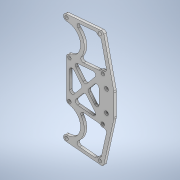
# Autodesk Inventor part: Knee_side_frame
Saved by Autodesk Inventor 2020.4 (Build 244396000, 396)
## iProperties
Created: 2021-09-05
Part Number: Knee_side_frame
Material: アルミニウム 2014-T4
Document SubType Name: Modeling
Designer: masato
Density: 2.8 g/cm^3
Appearance: 滑らか - 淡い灰色
Mass: 7.90232 g
Surface Area: 42.4892 cm^2
Volume: 2.82226 cm^3
Author: masato
Autodesk Inventor part; units mm, degrees
ref_plane "YZ Plane" through (0, 0, 0) normal (1, 0, 0) x (0, 1, 0)
ref_plane "XZ Plane" through (0, 0, 0) normal (0, 1, 0) x (-1, 0, 0)
ref_plane "XY Plane" through (0, 0, 0) normal (0, 0, 1) x (1, 0, 0)
sketch "スケッチ1" plane through (0, 0, 0) normal (0, 0, 1) x (1, 0, 0)
  line L0 (-32.2352, 43.3932) -> (10.6011, 47.1409) construction
  line L1 (10.6011, 47.1409) -> (13.3901, 15.2627) construction
  line L2 (13.3901, 15.2627) -> (-29.4462, 11.515) construction
  line L3 (-29.4462, 11.515) -> (-32.2352, 43.3932) construction
  line L4 (-32.2352, 43.3932) -> (13.3901, 15.2627) construction
  line L5 (10.6011, 47.1409) -> (-29.4462, 11.515) construction
  line L6 (-30.8407, 27.4541) -> (11.9956, 31.2018) construction
  line L7 (7.8305, 44.389) -> (-19.0668, 42.0358) construction
  line L8 (-19.0668, 42.0358) -> (-16.7136, 15.1385) construction
  line L9 (-16.7136, 15.1385) -> (10.1837, 17.4917) construction
  line L10 (10.1837, 17.4917) -> (7.8305, 44.389) construction
  line L11 (7.8305, 44.389) -> (-16.7136, 15.1385) construction
  line L12 (-19.0668, 42.0358) -> (10.1837, 17.4917) construction
  circle A0 centre (-18.8864, 28.5) radius 10.5 construction
  circle A1 centre (-19.0668, 42.0358) radius 1.35
  line L13 (-5.6182, 43.2124) -> (-3.265, 16.3151) construction
  circle A2 centre (7.8305, 44.389) radius 1.35
  circle A3 centre (-16.7136, 15.1385) radius 1.35
  circle A4 centre (10.1837, 17.4917) radius 1.35
  arc A5 (-21.4577, 41.8266) -> (-19.0348, 39.636) centre (-19.0668, 42.0358) ccw
  arc A6 (-17.0988, 17.5074) -> (-19.0348, 39.636) centre (-18.8864, 28.5) ccw
  arc A7 (-17.0988, 17.5074) -> (-19.1136, 15.1385) centre (-16.7136, 15.1385) ccw
  line L14 (-21.4577, 41.8266) -> (-21.6756, 44.3171)
  circle A8 centre (13.1136, 8.5) radius 1.55
  circle A9 centre (13.1136, 8.5) radius 6 construction
  circle A10 centre (13.1136, 8.5) radius 4.6 construction
  line L15 (19.1136, 8.5) -> (19.1136, -8.5)
  line L16 (-19.1136, 15.1385) -> (-19.1136, -15.1385)
  line L17 (-19.1136, 0) -> (19.1136, 0) construction
  line L18 (-21.6756, 44.3171) -> (10.6011, 47.1409)
  line L19 (10.6011, 47.1409) -> (18.9683, 9.8123)
  arc A11 (19.1136, 8.5) -> (18.9683, 9.8123) centre (13.1136, 8.5) ccw
  circle A12 centre (-18.8864, -28.5) radius 10.5 construction
  circle A13 centre (-19.0668, -42.0358) radius 1.35
  circle A14 centre (7.8305, -44.389) radius 1.35
  circle A15 centre (-16.7136, -15.1385) radius 1.35
  circle A16 centre (10.1837, -17.4917) radius 1.35
  arc A17 (-19.0348, -39.636) -> (-21.4577, -41.8266) centre (-19.0668, -42.0358) ccw
  arc A18 (-19.0348, -39.636) -> (-17.0988, -17.5074) centre (-18.8864, -28.5) ccw
  arc A19 (-19.1136, -15.1385) -> (-17.0988, -17.5074) centre (-16.7136, -15.1385) ccw
  line L20 (-21.4577, -41.8266) -> (-21.6756, -44.3171)
  circle A20 centre (13.1136, -8.5) radius 1.55
  circle A21 centre (13.1136, -8.5) radius 6 construction
  line L21 (-21.6756, -44.3171) -> (10.6011, -47.1409)
  line L22 (10.6011, -47.1409) -> (18.9683, -9.8123)
  arc A22 (18.9683, -9.8123) -> (19.1136, -8.5) centre (13.1136, -8.5) ccw
  line L23 (-16.7136, 15.1385) -> (10.1837, -17.4917) construction
  line L24 (-16.7136, -15.1385) -> (10.1837, 17.4917) construction
  line L25 (10.1837, -17.4917) -> (-16.7136, -15.1385) construction
  line L26 (-16.6136, 12.659) -> (-6.1788, 0)
  line L27 (-16.6136, 12.659) -> (-16.6136, -12.659)
  line L28 (-13.9357, 14.1268) -> (-4.2349, 2.3583)
  line L29 (-4.2349, 2.3583) -> (6.9739, 15.9561)
  line L30 (-13.9357, 14.1268) -> (6.9739, 15.9561)
  line L31 (-15.8832, 42.3143) -> (5.34, 44.1711)
  arc A23 (-10.7893, 16.9116) -> (-15.8832, 42.3143) centre (-18.8864, 28.5) ccw
  line L32 (-10.7893, 16.9116) -> (7.9179, 18.5483)
  line L33 (8.6713, 42.0346) -> (13.82, 19.0646)
  arc A24 (5.34, 44.1711) -> (8.6713, 42.0346) centre (7.8305, 44.389) ccw
  line L34 (-16.6136, -12.659) -> (-6.1788, 0)
  arc A25 (12.2315, 18.9257) -> (7.9179, 18.5483) centre (10.1837, 17.4917) ccw
  line L35 (12.2315, 18.9257) -> (13.82, 19.0646)
  line L36 (7.1136, 11.4091) -> (7.1136, -11.4091)
  line L37 (7.1136, 11.4091) -> (-2.2909, 0)
  line L38 (7.1136, -11.4091) -> (-2.2909, 0)
  line L39 (-13.9357, -14.1268) -> (-4.2349, -2.3583)
  line L40 (-4.2349, -2.3583) -> (6.9739, -15.9561)
  line L41 (-13.9357, -14.1268) -> (6.9739, -15.9561)
  line L42 (-15.8832, -42.3143) -> (5.34, -44.1711)
  arc A26 (-15.8832, -42.3143) -> (-10.7893, -16.9116) centre (-18.8864, -28.5) ccw
  line L43 (-10.7893, -16.9116) -> (7.9179, -18.5483)
  line L44 (8.6713, -42.0346) -> (13.82, -19.0646)
  arc A27 (8.6713, -42.0346) -> (5.34, -44.1711) centre (7.8305, -44.389) ccw
  arc A28 (7.9179, -18.5483) -> (12.2315, -18.9257) centre (10.1837, -17.4917) ccw
  line L45 (12.2315, -18.9257) -> (13.82, -19.0646)
  point P0 (0, 0)
  point P1 (-9.4225, 29.328)
  point P2 (-4.4416, 29.7638)
  dimension "d21" = 43
  dimension "d22" = 32
  dimension "d23" = 27
  dimension "d24" = 27
  dimension "d27" = 21
  dimension "d28" = 9.5
  dimension "d29" = 2.7
  dimension "d30" = 2.4
  dimension "d31" = 3.1
  dimension "d34" = 12
  dimension "d39" = 8.5
  dimension "d40" = 9.2
  dimension "d41" = 32
  dimension "d43" = 5
  dimension "d45" = 17
  dimension "d46" = 20
  dimension "d47" = 57
  dimension "d53" = 3
  dimension "d54" = 1.5
  dimension "d55" = 2.5
  dimension "d56" = 2.5
  dimension "d57" = 2.5
  dimension "d58" = 2.5
  dimension "d59" = 1.25
  dimension "d60" = 3
  dimension "d62" = 3
  dimension "d63" = 2.5
  dimension "d64" = 3
  dimension "d65" = 1.5
  constraints: 92 end point, 37 symmetric about line, 30 point on circle, 28 centre point, 14 parallel, 12 coincident, 12 midpoint, 6 tangent, 5 point on line, 4 perpendicular, 4 vertical, 1 collinear, 21 other
  measures "d21" distance of L1.end L2.end
  measures "d22" distance of L0.end L1.end
  measures "d23" distance of L9.end L8.end
  measures "d24" distance of L8.end L7.end
  measures "d27" diameter of A0
  measures "d28" distance of point (-9.423, 29.328) A0.centre
  measures "d29" diameter of A1
  measures "d30" radius of A5
  measures "d31" diameter of A8
  measures "d34" diameter of A9
  measures "d39" distance from line of L8 point (-9.423, 29.328)
  measures "d40" diameter of A10
  measures "d41" horizontal distance of A8.centre A0.centre
  measures "d43" angle of L17 L2
  measures "d45" distance of A20.centre A8.centre
  measures "d46" vertical distance of A11.centre A0.centre
  measures "d47" distance of A18.centre A0.centre
  measures "d53" distance between parallel lines of L26 L28
  measures "d54" distance between parallel lines of L23 L26
  measures "d55" distance between parallel lines of L16 L27
  measures "d56" radius of A24
  measures "d57" distance from line of L31.end L18
  measures "d58" distance between parallel lines of L32 L30
  measures "d59" distance between parallel lines of L30 L9
  measures "d60" radial gap between concentric circles of A23 A6
  measures "d62" distance between parallel lines of L19 L33
  measures "d63" radius of A25
  measures "d64" distance between parallel lines of L37 L29
  measures "d65" distance between parallel lines of L37 L24
extrude "押し出し1" add sketch "スケッチ1" along normal blind 2
fillet "フィレット1" radius 2 4 edges at (-21.6756, 44.3171, 1) (-21.6756, -44.3171, 1) (10.6011, -47.1409, 1) (10.6011, 47.1409, 1)
fillet "フィレット2" radius 2 26 edges at (-15.8832, 42.3143, 1) (-10.7893, 16.9116, 1) (13.82, 19.0646, 1) (12.2315, 18.9257, 1) (7.9179, 18.5483, 1) (5.34, 44.1711, 1) (8.6713, 42.0346, 1) (-13.9357, 14.1268, 1) (-16.6136, 12.659, 1) (-16.6136, -12.659, 1) (-6.1788, 0, 1) (-4.2349, 2.3583, 1) (-2.2909, 0, 1) (-13.9357, -14.1268, 1) (6.9739, -15.9561, 1) (7.1136, -11.4091, 1) (7.1136, 11.4091, 1) (6.9739, 15.9561, 1) (-10.7893, -16.9116, 1) (12.2315, -18.9257, 1) (13.82, -19.0646, 1) (7.9179, -18.5483, 1) (-15.8832, -42.3143, 1) (8.6713, -42.0346, 1) (5.34, -44.1711, 1) (-4.2349, -2.3583, 1)
